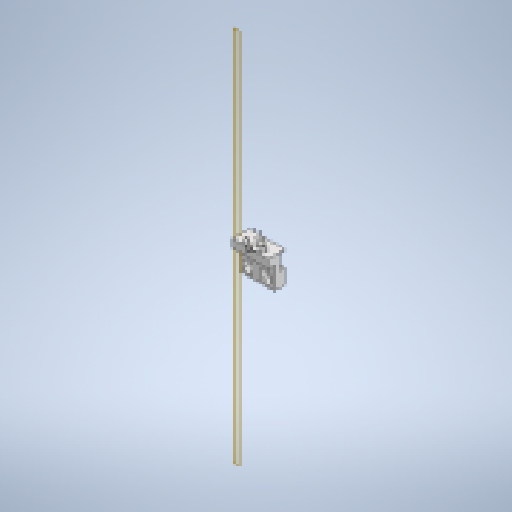
# Autodesk Inventor part: mountingPlate_V7
Saved by Autodesk Inventor 2023 (Build 270158000, 158)
## iProperties
Created: 2023-03-29
Part Number: mountingPlate_V7
Material: Generic
Document SubType Name: Modeling
Designer: shrey
Density: 1 g/cm^3
Appearance: Default
Author: shrey
Autodesk Inventor part; units mm, degrees
(part 1 of 3)
ref_plane "YZ Plane" through (0, 0, 0) normal (1, 0, 0) x (0, 1, 0)
ref_plane "XZ Plane" through (0, 0, 0) normal (0, 1, 0) x (-1, 0, 0)
ref_plane "XY Plane" through (0, 0, 0) normal (0, 0, 1) x (1, 0, 0)
ref_plane "Work Plane1" through (0, 0, 0) normal (0, 0, 1) x (-1, 0, 0)
sketch "Sketch2" plane through (0, 0, 0) normal (0, 0, 1) x (-1, 0, 0)
  spline S0 degree 3 poles (65.1879, 2.1547) (65.1796, 2.1356) (65.1474, 2.0656) (65.0811, 1.9497) (64.9926, 1.84) (64.9127, 1.7608) (64.8451, 1.7103) (64.7759, 1.6619) (64.6996, 1.6258) (64.6221, 1.5923) (64.54, 1.5725) (64.4573, 1.5558) (64.3447, 1.5518) (64.2044, 1.5544) (64.064, 1.5518) (63.9515, 1.5558) (63.8687, 1.5725) (63.7866, 1.5923) (63.7091, 1.6258) (63.6328, 1.6619) (63.5636, 1.7103) (63.4961, 1.7608) (63.4161, 1.84) (63.3277, 1.9497) (63.2437, 2.0964) (63.1793, 2.2524) (63.1317, 2.4143) (63.0866, 2.6344) (63.0241, 2.9083) (62.9282, 3.2316) (62.8191, 3.5506) (62.6977, 3.8651) (62.5657, 4.1753) (62.424, 4.4811) (62.2735, 4.7827) (62.1147, 5.08) (61.8936, 5.4714) (61.7138, 5.7566) (61.594, 5.9467) knots -0.66337 -0.66337 -0.66337 -0.66337 -0.657123 -0.640284 -0.623449 -0.615023 -0.606598 -0.598176 -0.589749 -0.581327 -0.572901 -0.564477 -0.556053 -0.5392 -0.522347 -0.513923 -0.505499 -0.497074 -0.488651 -0.480225 -0.471802 -0.463377 -0.454951 -0.438116 -0.421277 -0.40443 -0.387584 -0.370735 -0.337035 -0.303333 -0.26963 -0.235926 -0.202222 -0.168518 -0.134814 -0.101109 -0.067405 0 0 0 0 construction
  line L0 (61.594, 5.9467) -> (60.5318, 5.9467) construction
  spline S1 degree 3 poles (60.5318, 5.9467) (60.4119, 5.7566) (60.2321, 5.4714) (60.0111, 5.08) (59.8523, 4.7827) (59.7018, 4.4811) (59.5601, 4.1753) (59.428, 3.8651) (59.3066, 3.5506) (59.1976, 3.2316) (59.1016, 2.9083) (59.0392, 2.6344) (58.9941, 2.4143) (58.9464, 2.2524) (58.882, 2.0964) (58.7981, 1.9497) (58.7096, 1.84) (58.6297, 1.7608) (58.5621, 1.7103) (58.4929, 1.6619) (58.4166, 1.6258) (58.3391, 1.5923) (58.257, 1.5725) (58.1743, 1.5558) (58.0617, 1.5518) (57.9214, 1.5544) (57.781, 1.5518) (57.6685, 1.5558) (57.5857, 1.5725) (57.5036, 1.5923) (57.4261, 1.6258) (57.3498, 1.6619) (57.2806, 1.7103) (57.2131, 1.7608) (57.1331, 1.84) (57.0447, 1.9497) (56.9607, 2.0964) (56.8963, 2.2524) (56.8487, 2.4143) (56.8036, 2.6344) (56.7411, 2.9083) (56.6452, 3.2316) (56.5361, 3.5506) (56.4147, 3.8651) (56.2827, 4.1753) (56.141, 4.4811) (55.9905, 4.7827) (55.8317, 5.08) (55.6106, 5.4714) (55.4308, 5.7566) (55.311, 5.9467) knots -1.0784 -1.0784 -1.0784 -1.0784 -1.010995 -0.977291 -0.943586 -0.909882 -0.876178 -0.842474 -0.80877 -0.775067 -0.741365 -0.707665 -0.690816 -0.67397 -0.657123 -0.640284 -0.623449 -0.615023 -0.606598 -0.598176 -0.589749 -0.581327 -0.572901 -0.564477 -0.556053 -0.5392 -0.522347 -0.513923 -0.505499 -0.497074 -0.488651 -0.480225 -0.471802 -0.463377 -0.454951 -0.438116 -0.421277 -0.40443 -0.387584 -0.370735 -0.337035 -0.303333 -0.26963 -0.235926 -0.202222 -0.168518 -0.134814 -0.101109 -0.067405 0 0 0 0 construction
  line L1 (55.311, 5.9467) -> (54.2488, 5.9467) construction
  spline S2 degree 3 poles (54.2488, 5.9467) (54.1289, 5.7566) (53.9491, 5.4714) (53.7281, 5.08) (53.5693, 4.7827) (53.4188, 4.4811) (53.2771, 4.1753) (53.145, 3.8651) (53.0236, 3.5506) (52.9146, 3.2316) (52.8186, 2.9083) (52.7562, 2.6344) (52.7111, 2.4143) (52.6634, 2.2524) (52.599, 2.0964) (52.5151, 1.9497) (52.4266, 1.84) (52.3467, 1.7608) (52.2791, 1.7103) (52.2099, 1.6619) (52.1336, 1.6258) (52.0561, 1.5923) (51.974, 1.5725) (51.8913, 1.5558) (51.7787, 1.5518) (51.6384, 1.5544) (51.498, 1.5518) (51.3855, 1.5558) (51.3027, 1.5725) (51.2206, 1.5923) (51.1431, 1.6258) (51.0668, 1.6619) (50.9976, 1.7103) (50.9301, 1.7608) (50.8501, 1.84) (50.7617, 1.9497) (50.6777, 2.0964) (50.6133, 2.2524) (50.5657, 2.4143) (50.5206, 2.6344) (50.4581, 2.9083) (50.3622, 3.2316) (50.2531, 3.5506) (50.1317, 3.8651) (49.9997, 4.1753) (49.858, 4.4811) (49.7075, 4.7827) (49.5487, 5.08) (49.3276, 5.4714) (49.1478, 5.7566) (49.028, 5.9467) knots -1.0784 -1.0784 -1.0784 -1.0784 -1.010995 -0.977291 -0.943586 -0.909882 -0.876178 -0.842474 -0.80877 -0.775067 -0.741365 -0.707665 -0.690816 -0.67397 -0.657123 -0.640284 -0.623449 -0.615023 -0.606598 -0.598176 -0.589749 -0.581327 -0.572901 -0.564477 -0.556053 -0.5392 -0.522347 -0.513923 -0.505499 -0.497074 -0.488651 -0.480225 -0.471802 -0.463377 -0.454951 -0.438116 -0.421277 -0.40443 -0.387584 -0.370735 -0.337035 -0.303333 -0.26963 -0.235926 -0.202222 -0.168518 -0.134814 -0.101109 -0.067405 0 0 0 0 construction
  line L2 (49.028, 5.9467) -> (47.9658, 5.9467) construction
  spline S3 degree 3 poles (47.9658, 5.9467) (47.8459, 5.7566) (47.6661, 5.4714) (47.4451, 5.08) (47.2863, 4.7827) (47.1358, 4.4811) (46.9941, 4.1753) (46.862, 3.8651) (46.7406, 3.5506) (46.6316, 3.2316) (46.5356, 2.9083) (46.4732, 2.6344) (46.4281, 2.4143) (46.3804, 2.2524) (46.316, 2.0964) (46.2321, 1.9497) (46.1436, 1.84) (46.0637, 1.7608) (45.9961, 1.7103) (45.9269, 1.6619) (45.8506, 1.6258) (45.7731, 1.5923) (45.691, 1.5725) (45.6083, 1.5558) (45.4957, 1.5518) (45.3554, 1.5544) (45.215, 1.5518) (45.1025, 1.5558) (45.0197, 1.5725) (44.9376, 1.5923) (44.8601, 1.6258) (44.7838, 1.6619) (44.7146, 1.7103) (44.6471, 1.7608) (44.5671, 1.84) (44.4787, 1.9497) (44.3947, 2.0964) (44.3303, 2.2524) (44.2827, 2.4143) (44.2376, 2.6344) (44.1751, 2.9083) (44.0792, 3.2316) (43.9701, 3.5506) (43.8487, 3.8651) (43.7167, 4.1753) (43.575, 4.4811) (43.4245, 4.7827) (43.2657, 5.08) (43.0446, 5.4714) (42.8648, 5.7566) (42.745, 5.9467) knots -1.0784 -1.0784 -1.0784 -1.0784 -1.010995 -0.977291 -0.943586 -0.909882 -0.876178 -0.842474 -0.80877 -0.775067 -0.741365 -0.707665 -0.690816 -0.67397 -0.657123 -0.640284 -0.623449 -0.615023 -0.606598 -0.598176 -0.589749 -0.581327 -0.572901 -0.564477 -0.556053 -0.5392 -0.522347 -0.513923 -0.505499 -0.497074 -0.488651 -0.480225 -0.471802 -0.463377 -0.454951 -0.438116 -0.421277 -0.40443 -0.387584 -0.370735 -0.337035 -0.303333 -0.26963 -0.235926 -0.202222 -0.168518 -0.134814 -0.101109 -0.067405 0 0 0 0 construction
  line L3 (42.745, 5.9467) -> (41.6828, 5.9467) construction
  spline S4 degree 3 poles (41.6828, 5.9467) (41.5629, 5.7566) (41.3831, 5.4714) (41.1621, 5.08) (41.0033, 4.7827) (40.8528, 4.4811) (40.7111, 4.1753) (40.579, 3.8651) (40.4576, 3.5506) (40.3486, 3.2316) (40.2526, 2.9083) (40.1902, 2.6344) (40.1451, 2.4143) (40.0974, 2.2524) (40.033, 2.0964) (39.9491, 1.9497) (39.8606, 1.84) (39.7807, 1.7608) (39.7131, 1.7103) (39.6439, 1.6619) (39.5676, 1.6258) (39.4901, 1.5923) (39.408, 1.5725) (39.3253, 1.5558) (39.2127, 1.5518) (39.0724, 1.5544) (38.932, 1.5518) (38.8195, 1.5558) (38.7367, 1.5725) (38.6546, 1.5923) (38.5771, 1.6258) (38.5008, 1.6619) (38.4316, 1.7103) (38.3641, 1.7608) (38.2841, 1.84) (38.1957, 1.9497) (38.1117, 2.0964) (38.0473, 2.2524) (37.9997, 2.4143) (37.9546, 2.6344) (37.8921, 2.9083) (37.7962, 3.2316) (37.6871, 3.5506) (37.5657, 3.8651) (37.4337, 4.1753) (37.292, 4.4811) (37.1415, 4.7827) (36.9827, 5.08) (36.7616, 5.4714) (36.5818, 5.7566) (36.462, 5.9467) knots -1.0784 -1.0784 -1.0784 -1.0784 -1.010995 -0.977291 -0.943586 -0.909882 -0.876178 -0.842474 -0.80877 -0.775067 -0.741365 -0.707665 -0.690816 -0.67397 -0.657123 -0.640284 -0.623449 -0.615023 -0.606598 -0.598176 -0.589749 -0.581327 -0.572901 -0.564477 -0.556053 -0.5392 -0.522347 -0.513923 -0.505499 -0.497074 -0.488651 -0.480225 -0.471802 -0.463377 -0.454951 -0.438116 -0.421277 -0.40443 -0.387584 -0.370735 -0.337035 -0.303333 -0.26963 -0.235926 -0.202222 -0.168518 -0.134814 -0.101109 -0.067405 0 0 0 0 construction
  line L4 (36.462, 5.9467) -> (35.3998, 5.9467) construction
  spline S5 degree 3 poles (35.3998, 5.9467) (35.2799, 5.7566) (35.1001, 5.4714) (34.8791, 5.08) (34.7203, 4.7827) (34.5698, 4.4811) (34.4281, 4.1753) (34.296, 3.8651) (34.1746, 3.5506) (34.0656, 3.2316) (33.9696, 2.9083) (33.9072, 2.6344) (33.8621, 2.4143) (33.8144, 2.2524) (33.75, 2.0964) (33.6661, 1.9497) (33.5776, 1.84) (33.4977, 1.7608) (33.4301, 1.7103) (33.3609, 1.6619) (33.2846, 1.6258) (33.2071, 1.5923) (33.125, 1.5725) (33.0423, 1.5558) (32.9297, 1.5518) (32.7894, 1.5544) (32.649, 1.5518) (32.5365, 1.5558) (32.4537, 1.5725) (32.3716, 1.5923) (32.2941, 1.6258) (32.2178, 1.6619) (32.1486, 1.7103) (32.0811, 1.7608) (32.0011, 1.84) (31.9127, 1.9497) (31.8287, 2.0964) (31.7643, 2.2524) (31.7167, 2.4143) (31.6716, 2.6344) (31.6091, 2.9083) (31.5132, 3.2316) (31.4041, 3.5506) (31.2827, 3.8651) (31.1507, 4.1753) (31.009, 4.4811) (30.8585, 4.7827) (30.6997, 5.08) (30.4786, 5.4714) (30.2988, 5.7566) (30.179, 5.9467) knots -1.0784 -1.0784 -1.0784 -1.0784 -1.010995 -0.977291 -0.943586 -0.909882 -0.876178 -0.842474 -0.80877 -0.775067 -0.741365 -0.707665 -0.690816 -0.67397 -0.657123 -0.640284 -0.623449 -0.615023 -0.606598 -0.598176 -0.589749 -0.581327 -0.572901 -0.564477 -0.556053 -0.5392 -0.522347 -0.513923 -0.505499 -0.497074 -0.488651 -0.480225 -0.471802 -0.463377 -0.454951 -0.438116 -0.421277 -0.40443 -0.387584 -0.370735 -0.337035 -0.303333 -0.26963 -0.235926 -0.202222 -0.168518 -0.134814 -0.101109 -0.067405 0 0 0 0 construction
  line L5 (30.179, 5.9467) -> (29.1168, 5.9467) construction
  spline S6 degree 3 poles (29.1168, 5.9467) (28.9969, 5.7566) (28.8171, 5.4714) (28.5961, 5.08) (28.4373, 4.7827) (28.2868, 4.4811) (28.1451, 4.1753) (28.013, 3.8651) (27.8916, 3.5506) (27.7826, 3.2316) (27.6866, 2.9083) (27.6242, 2.6344) (27.5791, 2.4143) (27.5314, 2.2524) (27.467, 2.0964) (27.3831, 1.9497) (27.2946, 1.84) (27.2147, 1.7608) (27.1471, 1.7103) (27.0779, 1.6619) (27.0016, 1.6258) (26.9241, 1.5923) (26.842, 1.5725) (26.7593, 1.5558) (26.6467, 1.5518) (26.5064, 1.5544) (26.366, 1.5518) (26.2535, 1.5558) (26.1707, 1.5725) (26.0886, 1.5923) (26.0111, 1.6258) (25.9348, 1.6619) (25.8656, 1.7103) (25.7981, 1.7608) (25.7181, 1.84) (25.6297, 1.9497) (25.5457, 2.0964) (25.4813, 2.2524) (25.4337, 2.4143) (25.3886, 2.6344) (25.3261, 2.9083) (25.2302, 3.2316) (25.1211, 3.5506) (24.9997, 3.8651) (24.8677, 4.1753) (24.726, 4.4811) (24.5755, 4.7827) (24.4167, 5.08) (24.1956, 5.4714) (24.0158, 5.7566) (23.896, 5.9467) knots -1.0784 -1.0784 -1.0784 -1.0784 -1.010995 -0.977291 -0.943586 -0.909882 -0.876178 -0.842474 -0.80877 -0.775067 -0.741365 -0.707665 -0.690816 -0.67397 -0.657123 -0.640284 -0.623449 -0.615023 -0.606598 -0.598176 -0.589749 -0.581327 -0.572901 -0.564477 -0.556053 -0.5392 -0.522347 -0.513923 -0.505499 -0.497074 -0.488651 -0.480225 -0.471802 -0.463377 -0.454951 -0.438116 -0.421277 -0.40443 -0.387584 -0.370735 -0.337035 -0.303333 -0.26963 -0.235926 -0.202222 -0.168518 -0.134814 -0.101109 -0.067405 0 0 0 0 construction
  line L6 (23.896, 5.9467) -> (22.8338, 5.9467) construction
  spline S7 degree 3 poles (22.8338, 5.9467) (22.7139, 5.7566) (22.5341, 5.4714) (22.3131, 5.08) (22.1543, 4.7827) (22.0038, 4.4811) (21.8621, 4.1753) (21.73, 3.8651) (21.6086, 3.5506) (21.4996, 3.2316) (21.4036, 2.9083) (21.3412, 2.6344) (21.2961, 2.4143) (21.2484, 2.2524) (21.184, 2.0964) (21.1001, 1.9497) (21.0116, 1.84) (20.9317, 1.7608) (20.8641, 1.7103) (20.7949, 1.6619) (20.7186, 1.6258) (20.6411, 1.5923) (20.559, 1.5725) (20.4763, 1.5558) (20.3637, 1.5518) (20.2234, 1.5544) (20.083, 1.5518) (19.9705, 1.5558) (19.8877, 1.5725) (19.8056, 1.5923) (19.7281, 1.6258) (19.6518, 1.6619) (19.5826, 1.7103) (19.5151, 1.7608) (19.4351, 1.84) (19.3467, 1.9497) (19.2627, 2.0964) (19.1983, 2.2524) (19.1507, 2.4143) (19.1056, 2.6344) (19.0431, 2.9083) (18.9472, 3.2316) (18.8381, 3.5506) (18.7167, 3.8651) (18.5847, 4.1753) (18.443, 4.4811) (18.2925, 4.7827) (18.1337, 5.08) (17.9126, 5.4714) (17.7328, 5.7566) (17.613, 5.9467) knots -1.0784 -1.0784 -1.0784 -1.0784 -1.010995 -0.977291 -0.943586 -0.909882 -0.876178 -0.842474 -0.80877 -0.775067 -0.741365 -0.707665 -0.690816 -0.67397 -0.657123 -0.640284 -0.623449 -0.615023 -0.606598 -0.598176 -0.589749 -0.581327 -0.572901 -0.564477 -0.556053 -0.5392 -0.522347 -0.513923 -0.505499 -0.497074 -0.488651 -0.480225 -0.471802 -0.463377 -0.454951 -0.438116 -0.421277 -0.40443 -0.387584 -0.370735 -0.337035 -0.303333 -0.26963 -0.235926 -0.202222 -0.168518 -0.134814 -0.101109 -0.067405 0 0 0 0 construction
  line L7 (17.613, 5.9467) -> (16.5508, 5.9467) construction
  spline S8 degree 3 poles (16.5508, 5.9467) (16.4309, 5.7566) (16.2511, 5.4714) (16.0301, 5.08) (15.8713, 4.7827) (15.7208, 4.4811) (15.5791, 4.1753) (15.447, 3.8651) (15.3256, 3.5506) (15.2166, 3.2316) (15.1206, 2.9083) (15.0582, 2.6344) (15.0131, 2.4143) (14.9654, 2.2524) (14.901, 2.0964) (14.8171, 1.9497) (14.7286, 1.84) (14.6487, 1.7608) (14.5811, 1.7103) (14.5119, 1.6619) (14.4356, 1.6258) (14.3581, 1.5923) (14.276, 1.5725) (14.1933, 1.5558) (14.0807, 1.5518) (13.9404, 1.5544) (13.8, 1.5518) (13.6875, 1.5558) (13.6047, 1.5725) (13.5226, 1.5923) (13.4451, 1.6258) (13.3688, 1.6619) (13.2996, 1.7103) (13.2321, 1.7608) (13.1521, 1.84) (13.0637, 1.9497) (12.9797, 2.0964) (12.9153, 2.2524) (12.8677, 2.4143) (12.8226, 2.6344) (12.7601, 2.9083) (12.6642, 3.2316) (12.5551, 3.5506) (12.4337, 3.8651) (12.3017, 4.1753) (12.16, 4.4811) (12.0095, 4.7827) (11.8507, 5.08) (11.6296, 5.4714) (11.4498, 5.7566) (11.33, 5.9467) knots -1.0784 -1.0784 -1.0784 -1.0784 -1.010995 -0.977291 -0.943586 -0.909882 -0.876178 -0.842474 -0.80877 -0.775067 -0.741365 -0.707665 -0.690816 -0.67397 -0.657123 -0.640284 -0.623449 -0.615023 -0.606598 -0.598176 -0.589749 -0.581327 -0.572901 -0.564477 -0.556053 -0.5392 -0.522347 -0.513923 -0.505499 -0.497074 -0.488651 -0.480225 -0.471802 -0.463377 -0.454951 -0.438116 -0.421277 -0.40443 -0.387584 -0.370735 -0.337035 -0.303333 -0.26963 -0.235926 -0.202222 -0.168518 -0.134814 -0.101109 -0.067405 0 0 0 0 construction
  line L8 (11.33, 5.9467) -> (10.2678, 5.9467) construction
  spline S9 degree 3 poles (10.2678, 5.9467) (10.1479, 5.7566) (9.9681, 5.4714) (9.7471, 5.08) (9.5883, 4.7827) (9.4378, 4.4811) (9.2961, 4.1753) (9.164, 3.8651) (9.0426, 3.5506) (8.9336, 3.2316) (8.8376, 2.9083) (8.7752, 2.6344) (8.7301, 2.4143) (8.6824, 2.2524) (8.618, 2.0964) (8.5341, 1.9497) (8.4456, 1.84) (8.3657, 1.7608) (8.2981, 1.7103) (8.2289, 1.6619) (8.1526, 1.6258) (8.0751, 1.5923) (7.993, 1.5725) (7.9103, 1.5558) (7.7977, 1.5518) (7.6574, 1.5544) (7.517, 1.5518) (7.4045, 1.5558) (7.3217, 1.5725) (7.2396, 1.5923) (7.1621, 1.6258) (7.0858, 1.6619) (7.0166, 1.7103) (6.9491, 1.7608) (6.8691, 1.84) (6.7807, 1.9497) (6.6967, 2.0964) (6.6323, 2.2524) (6.5847, 2.4143) (6.5396, 2.6344) (6.4771, 2.9083) (6.3812, 3.2316) (6.2721, 3.5506) (6.1507, 3.8651) (6.0187, 4.1753) (5.877, 4.4811) (5.7265, 4.7827) (5.5677, 5.08) (5.3466, 5.4714) (5.1668, 5.7566) (5.047, 5.9467) knots -1.0784 -1.0784 -1.0784 -1.0784 -1.010995 -0.977291 -0.943586 -0.909882 -0.876178 -0.842474 -0.80877 -0.775067 -0.741365 -0.707665 -0.690816 -0.67397 -0.657123 -0.640284 -0.623449 -0.615023 -0.606598 -0.598176 -0.589749 -0.581327 -0.572901 -0.564477 -0.556053 -0.5392 -0.522347 -0.513923 -0.505499 -0.497074 -0.488651 -0.480225 -0.471802 -0.463377 -0.454951 -0.438116 -0.421277 -0.40443 -0.387584 -0.370735 -0.337035 -0.303333 -0.26963 -0.235926 -0.202222 -0.168518 -0.134814 -0.101109 -0.067405 0 0 0 0 construction
  line L9 (5.047, 5.9467) -> (3.9848, 5.9467) construction
  spline S10 degree 3 poles (3.9848, 5.9467) (3.8649, 5.7566) (3.6851, 5.4714) (3.4641, 5.08) (3.3053, 4.7827) (3.1548, 4.4811) (3.0131, 4.1753) (2.881, 3.8651) (2.7596, 3.5506) (2.6506, 3.2316) (2.5546, 2.9083) (2.4922, 2.6344) (2.4471, 2.4143) (2.3994, 2.2524) (2.335, 2.0964) (2.2511, 1.9497) (2.1626, 1.84) (2.0827, 1.7608) (2.0151, 1.7103) (1.9459, 1.6619) (1.8696, 1.6258) (1.7921, 1.5923) (1.71, 1.5725) (1.6273, 1.5558) (1.5147, 1.5518) (1.3744, 1.5544) (1.234, 1.5518) (1.1215, 1.5558) (1.0387, 1.5725) (0.9566, 1.5923) (0.8791, 1.6258) (0.8028, 1.6619) (0.7336, 1.7103) (0.6661, 1.7608) (0.5861, 1.84) (0.4977, 1.9497) (0.4137, 2.0964) (0.3493, 2.2524) (0.3017, 2.4143) (0.2566, 2.6344) (0.1941, 2.9083) (0.0982, 3.2316) (-0.0109, 3.5506) (-0.1323, 3.8651) (-0.2643, 4.1753) (-0.406, 4.4811) (-0.5565, 4.7827) (-0.7153, 5.08) (-0.9364, 5.4714) (-1.1162, 5.7566) (-1.236, 5.9467) knots -1.0784 -1.0784 -1.0784 -1.0784 -1.010995 -0.977291 -0.943586 -0.909882 -0.876178 -0.842474 -0.80877 -0.775067 -0.741365 -0.707665 -0.690816 -0.67397 -0.657123 -0.640284 -0.623449 -0.615023 -0.606598 -0.598176 -0.589749 -0.581327 -0.572901 -0.564477 -0.556053 -0.5392 -0.522347 -0.513923 -0.505499 -0.497074 -0.488651 -0.480225 -0.471802 -0.463377 -0.454951 -0.438116 -0.421277 -0.40443 -0.387584 -0.370735 -0.337035 -0.303333 -0.26963 -0.235926 -0.202222 -0.168518 -0.134814 -0.101109 -0.067405 0 0 0 0 construction
  line L10 (-1.236, 5.9467) -> (-2.2982, 5.9467) construction
  spline S11 degree 3 poles (-2.2982, 5.9467) (-2.4181, 5.7566) (-2.5979, 5.4714) (-2.8189, 5.08) (-2.9777, 4.7827) (-3.1282, 4.4811) (-3.2699, 4.1753) (-3.402, 3.8651) (-3.5234, 3.5506) (-3.6324, 3.2316) (-3.7284, 2.9083) (-3.7908, 2.6344) (-3.8359, 2.4143) (-3.8836, 2.2524) (-3.948, 2.0964) (-4.0319, 1.9497) (-4.1204, 1.84) (-4.2003, 1.7608) (-4.2679, 1.7103) (-4.3371, 1.6619) (-4.4134, 1.6258) (-4.4909, 1.5923) (-4.573, 1.5725) (-4.6557, 1.5558) (-4.7683, 1.5518) (-4.9086, 1.5544) (-5.049, 1.5518) (-5.1615, 1.5558) (-5.2443, 1.5725) (-5.3264, 1.5923) (-5.4039, 1.6258) (-5.4802, 1.6619) (-5.5494, 1.7103) (-5.6169, 1.7608) (-5.6969, 1.84) (-5.7853, 1.9497) (-5.8693, 2.0964) (-5.9337, 2.2524) (-5.9813, 2.4143) (-6.0264, 2.6344) (-6.0889, 2.9083) (-6.1848, 3.2316) (-6.2939, 3.5506) (-6.4153, 3.8651) (-6.5473, 4.1753) (-6.689, 4.4811) (-6.8395, 4.7827) (-6.9983, 5.08) (-7.2194, 5.4714) (-7.3992, 5.7566) (-7.519, 5.9467) knots -1.0784 -1.0784 -1.0784 -1.0784 -1.010995 -0.977291 -0.943586 -0.909882 -0.876178 -0.842474 -0.80877 -0.775067 -0.741365 -0.707665 -0.690816 -0.67397 -0.657123 -0.640284 -0.623449 -0.615023 -0.606598 -0.598176 -0.589749 -0.581327 -0.572901 -0.564477 -0.556053 -0.5392 -0.522347 -0.513923 -0.505499 -0.497074 -0.488651 -0.480225 -0.471802 -0.463377 -0.454951 -0.438116 -0.421277 -0.40443 -0.387584 -0.370735 -0.337035 -0.303333 -0.26963 -0.235926 -0.202222 -0.168518 -0.134814 -0.101109 -0.067405 0 0 0 0 construction
  line L11 (-7.519, 5.9467) -> (-8.5812, 5.9467) construction
  spline S12 degree 3 poles (-8.5812, 5.9467) (-8.7011, 5.7566) (-8.8809, 5.4714) (-9.1019, 5.08) (-9.2607, 4.7827) (-9.4112, 4.4811) (-9.5529, 4.1753) (-9.685, 3.8651) (-9.8064, 3.5506) (-9.9154, 3.2316) (-10.0114, 2.9083) (-10.0738, 2.6344) (-10.1189, 2.4143) (-10.1666, 2.2524) (-10.231, 2.0964) (-10.3149, 1.9497) (-10.4034, 1.84) (-10.4833, 1.7608) (-10.5509, 1.7103) (-10.6201, 1.6619) (-10.6964, 1.6258) (-10.7739, 1.5923) (-10.856, 1.5725) (-10.9387, 1.5558) (-11.0513, 1.5518) (-11.1916, 1.5544) (-11.332, 1.5518) (-11.4445, 1.5558) (-11.5273, 1.5725) (-11.6094, 1.5923) (-11.6869, 1.6258) (-11.7632, 1.6619) (-11.8324, 1.7103) (-11.8999, 1.7608) (-11.9799, 1.84) (-12.0683, 1.9497) (-12.1523, 2.0964) (-12.2167, 2.2524) (-12.2643, 2.4143) (-12.3094, 2.6344) (-12.3719, 2.9083) (-12.4678, 3.2316) (-12.5769, 3.5506) (-12.6983, 3.8651) (-12.8303, 4.1753) (-12.972, 4.4811) (-13.1225, 4.7827) (-13.2813, 5.08) (-13.5024, 5.4714) (-13.6822, 5.7566) (-13.802, 5.9467) knots -1.0784 -1.0784 -1.0784 -1.0784 -1.010995 -0.977291 -0.943586 -0.909882 -0.876178 -0.842474 -0.80877 -0.775067 -0.741365 -0.707665 -0.690816 -0.67397 -0.657123 -0.640284 -0.623449 -0.615023 -0.606598 -0.598176 -0.589749 -0.581327 -0.572901 -0.564477 -0.556053 -0.5392 -0.522347 -0.513923 -0.505499 -0.497074 -0.488651 -0.480225 -0.471802 -0.463377 -0.454951 -0.438116 -0.421277 -0.40443 -0.387584 -0.370735 -0.337035 -0.303333 -0.26963 -0.235926 -0.202222 -0.168518 -0.134814 -0.101109 -0.067405 0 0 0 0 construction
  line L12 (-13.802, 5.9467) -> (-14.8642, 5.9467) construction
  spline S13 degree 3 poles (-14.8642, 5.9467) (-14.9841, 5.7566) (-15.1639, 5.4714) (-15.3849, 5.08) (-15.5437, 4.7827) (-15.6942, 4.4811) (-15.8359, 4.1753) (-15.968, 3.8651) (-16.0894, 3.5506) (-16.1984, 3.2316) (-16.2944, 2.9083) (-16.3568, 2.6344) (-16.4019, 2.4143) (-16.4496, 2.2524) (-16.514, 2.0964) (-16.5979, 1.9497) (-16.6864, 1.84) (-16.7663, 1.7608) (-16.8339, 1.7103) (-16.9031, 1.6619) (-16.9794, 1.6258) (-17.0569, 1.5923) (-17.139, 1.5725) (-17.2217, 1.5558) (-17.3343, 1.5518) (-17.4746, 1.5544) (-17.615, 1.5518) (-17.7275, 1.5558) (-17.8103, 1.5725) (-17.8924, 1.5923) (-17.9699, 1.6258) (-18.0462, 1.6619) (-18.1154, 1.7103) (-18.1829, 1.7608) (-18.2629, 1.84) (-18.3513, 1.9497) (-18.4353, 2.0964) (-18.4997, 2.2524) (-18.5473, 2.4143) (-18.5924, 2.6344) (-18.6549, 2.9083) (-18.7508, 3.2316) (-18.8599, 3.5506) (-18.9813, 3.8651) (-19.1133, 4.1753) (-19.255, 4.4811) (-19.4055, 4.7827) (-19.5643, 5.08) (-19.7854, 5.4714) (-19.9652, 5.7566) (-20.085, 5.9467) knots -1.0784 -1.0784 -1.0784 -1.0784 -1.010995 -0.977291 -0.943586 -0.909882 -0.876178 -0.842474 -0.80877 -0.775067 -0.741365 -0.707665 -0.690816 -0.67397 -0.657123 -0.640284 -0.623449 -0.615023 -0.606598 -0.598176 -0.589749 -0.581327 -0.572901 -0.564477 -0.556053 -0.5392 -0.522347 -0.513923 -0.505499 -0.497074 -0.488651 -0.480225 -0.471802 -0.463377 -0.454951 -0.438116 -0.421277 -0.40443 -0.387584 -0.370735 -0.337035 -0.303333 -0.26963 -0.235926 -0.202222 -0.168518 -0.134814 -0.101109 -0.067405 0 0 0 0 construction
  line L13 (-20.085, 5.9467) -> (-21.1472, 5.9467) construction
  spline S14 degree 3 poles (-21.1472, 5.9467) (-21.2671, 5.7566) (-21.4469, 5.4714) (-21.6679, 5.08) (-21.8267, 4.7827) (-21.9772, 4.4811) (-22.1189, 4.1753) (-22.251, 3.8651) (-22.3724, 3.5506) (-22.4814, 3.2316) (-22.5774, 2.9083) (-22.6398, 2.6344) (-22.6849, 2.4143) (-22.7326, 2.2524) (-22.797, 2.0964) (-22.8809, 1.9497) (-22.9694, 1.84) (-23.0493, 1.7608) (-23.1169, 1.7103) (-23.1861, 1.6619) (-23.2624, 1.6258) (-23.3399, 1.5923) (-23.422, 1.5725) (-23.5047, 1.5558) (-23.6173, 1.5518) (-23.7576, 1.5544) (-23.898, 1.5518) (-24.0105, 1.5558) (-24.0933, 1.5725) (-24.1754, 1.5923) (-24.2529, 1.6258) (-24.3292, 1.6619) (-24.3984, 1.7103) (-24.4659, 1.7608) (-24.5459, 1.84) (-24.6343, 1.9497) (-24.7183, 2.0964) (-24.7827, 2.2524) (-24.8303, 2.4143) (-24.8754, 2.6344) (-24.9379, 2.9083) (-25.0338, 3.2316) (-25.1429, 3.5506) (-25.2643, 3.8651) (-25.3963, 4.1753) (-25.538, 4.4811) (-25.6885, 4.7827) (-25.8473, 5.08) (-26.0684, 5.4714) (-26.2482, 5.7566) (-26.368, 5.9467) knots -1.0784 -1.0784 -1.0784 -1.0784 -1.010995 -0.977291 -0.943586 -0.909882 -0.876178 -0.842474 -0.80877 -0.775067 -0.741365 -0.707665 -0.690816 -0.67397 -0.657123 -0.640284 -0.623449 -0.615023 -0.606598 -0.598176 -0.589749 -0.581327 -0.572901 -0.564477 -0.556053 -0.5392 -0.522347 -0.513923 -0.505499 -0.497074 -0.488651 -0.480225 -0.471802 -0.463377 -0.454951 -0.438116 -0.421277 -0.40443 -0.387584 -0.370735 -0.337035 -0.303333 -0.26963 -0.235926 -0.202222 -0.168518 -0.134814 -0.101109 -0.067405 0 0 0 0 construction
  line L14 (-26.368, 5.9467) -> (-27.4302, 5.9467) construction
  spline S15 degree 3 poles (-27.4302, 5.9467) (-27.5501, 5.7566) (-27.7299, 5.4714) (-27.9509, 5.08) (-28.1097, 4.7827) (-28.2602, 4.4811) (-28.4019, 4.1753) (-28.534, 3.8651) (-28.6554, 3.5506) (-28.7644, 3.2316) (-28.8604, 2.9083) (-28.9228, 2.6344) (-28.9679, 2.4143) (-29.0156, 2.2524) (-29.08, 2.0964) (-29.1639, 1.9497) (-29.2524, 1.84) (-29.3323, 1.7608) (-29.3999, 1.7103) (-29.4691, 1.6619) (-29.5454, 1.6258) (-29.6229, 1.5923) (-29.705, 1.5725) (-29.7877, 1.5558) (-29.9003, 1.5518) (-30.0406, 1.5544) (-30.181, 1.5518) (-30.2935, 1.5558) (-30.3763, 1.5725) (-30.4584, 1.5923) (-30.5359, 1.6258) (-30.6122, 1.6619) (-30.6814, 1.7103) (-30.7489, 1.7608) (-30.8289, 1.84) (-30.9173, 1.9497) (-31.0013, 2.0964) (-31.0657, 2.2524) (-31.1133, 2.4143) (-31.1584, 2.6344) (-31.2209, 2.9083) (-31.3168, 3.2316) (-31.4259, 3.5506) (-31.5473, 3.8651) (-31.6793, 4.1753) (-31.821, 4.4811) (-31.9715, 4.7827) (-32.1303, 5.08) (-32.3514, 5.4714) (-32.5312, 5.7566) (-32.651, 5.9467) knots -1.0784 -1.0784 -1.0784 -1.0784 -1.010995 -0.977291 -0.943586 -0.909882 -0.876178 -0.842474 -0.80877 -0.775067 -0.741365 -0.707665 -0.690816 -0.67397 -0.657123 -0.640284 -0.623449 -0.615023 -0.606598 -0.598176 -0.589749 -0.581327 -0.572901 -0.564477 -0.556053 -0.5392 -0.522347 -0.513923 -0.505499 -0.497074 -0.488651 -0.480225 -0.471802 -0.463377 -0.454951 -0.438116 -0.421277 -0.40443 -0.387584 -0.370735 -0.337035 -0.303333 -0.26963 -0.235926 -0.202222 -0.168518 -0.134814 -0.101109 -0.067405 0 0 0 0 construction
  line L15 (-32.651, 5.9467) -> (-33.7132, 5.9467) construction
  spline S16 degree 3 poles (-33.7132, 5.9467) (-33.8331, 5.7566) (-34.0129, 5.4714) (-34.2339, 5.08) (-34.3927, 4.7827) (-34.5432, 4.4811) (-34.6849, 4.1753) (-34.817, 3.8651) (-34.9384, 3.5506) (-35.0474, 3.2316) (-35.1434, 2.9083) (-35.2058, 2.6344) (-35.2509, 2.4143) (-35.2986, 2.2524) (-35.363, 2.0964) (-35.4469, 1.9497) (-35.5354, 1.84) (-35.6153, 1.7608) (-35.6829, 1.7103) (-35.7521, 1.6619) (-35.8284, 1.6258) (-35.9059, 1.5923) (-35.988, 1.5725) (-36.0707, 1.5558) (-36.1833, 1.5518) (-36.3236, 1.5544) (-36.464, 1.5518) (-36.5765, 1.5558) (-36.6593, 1.5725) (-36.7414, 1.5923) (-36.8189, 1.6258) (-36.8952, 1.6619) (-36.9644, 1.7103) (-37.0319, 1.7608) (-37.1119, 1.84) (-37.2003, 1.9497) (-37.2843, 2.0964) (-37.3487, 2.2524) (-37.3963, 2.4143) (-37.4414, 2.6344) (-37.5039, 2.9083) (-37.5998, 3.2316) (-37.7089, 3.5506) (-37.8303, 3.8651) (-37.9623, 4.1753) (-38.104, 4.4811) (-38.2545, 4.7827) (-38.4133, 5.08) (-38.6344, 5.4714) (-38.8142, 5.7566) (-38.934, 5.9467) knots -1.0784 -1.0784 -1.0784 -1.0784 -1.010995 -0.977291 -0.943586 -0.909882 -0.876178 -0.842474 -0.80877 -0.775067 -0.741365 -0.707665 -0.690816 -0.67397 -0.657123 -0.640284 -0.623449 -0.615023 -0.606598 -0.598176 -0.589749 -0.581327 -0.572901 -0.564477 -0.556053 -0.5392 -0.522347 -0.513923 -0.505499 -0.497074 -0.488651 -0.480225 -0.471802 -0.463377 -0.454951 -0.438116 -0.421277 -0.40443 -0.387584 -0.370735 -0.337035 -0.303333 -0.26963 -0.235926 -0.202222 -0.168518 -0.134814 -0.101109 -0.067405 0 0 0 0 construction
  line L16 (-38.934, 5.9467) -> (-39.9962, 5.9467) construction
  spline S17 degree 3 poles (-39.9962, 5.9467) (-40.1161, 5.7566) (-40.2959, 5.4714) (-40.5169, 5.08) (-40.6757, 4.7827) (-40.8262, 4.4811) (-40.9679, 4.1753) (-41.1, 3.8651) (-41.2214, 3.5506) (-41.3304, 3.2316) (-41.4264, 2.9083) (-41.4888, 2.6344) (-41.5339, 2.4143) (-41.5816, 2.2524) (-41.646, 2.0964) (-41.7299, 1.9497) (-41.8184, 1.84) (-41.8983, 1.7608) (-41.9659, 1.7103) (-42.0351, 1.6619) (-42.1114, 1.6258) (-42.1889, 1.5923) (-42.271, 1.5725) (-42.3537, 1.5558) (-42.4663, 1.5518) (-42.6066, 1.5544) (-42.747, 1.5518) (-42.8595, 1.5558) (-42.9423, 1.5725) (-43.0244, 1.5923) (-43.1019, 1.6258) (-43.1782, 1.6619) (-43.2474, 1.7103) (-43.3149, 1.7608) (-43.3949, 1.84) (-43.4833, 1.9497) (-43.5673, 2.0964) (-43.6317, 2.2524) (-43.6793, 2.4143) (-43.7244, 2.6344) (-43.7869, 2.9083) (-43.8828, 3.2316) (-43.9919, 3.5506) (-44.1133, 3.8651) (-44.2453, 4.1753) (-44.387, 4.4811) (-44.5375, 4.7827) (-44.6963, 5.08) (-44.9174, 5.4714) (-45.0972, 5.7566) (-45.217, 5.9467) knots -1.0784 -1.0784 -1.0784 -1.0784 -1.010995 -0.977291 -0.943586 -0.909882 -0.876178 -0.842474 -0.80877 -0.775067 -0.741365 -0.707665 -0.690816 -0.67397 -0.657123 -0.640284 -0.623449 -0.615023 -0.606598 -0.598176 -0.589749 -0.581327 -0.572901 -0.564477 -0.556053 -0.5392 -0.522347 -0.513923 -0.505499 -0.497074 -0.488651 -0.480225 -0.471802 -0.463377 -0.454951 -0.438116 -0.421277 -0.40443 -0.387584 -0.370735 -0.337035 -0.303333 -0.26963 -0.235926 -0.202222 -0.168518 -0.134814 -0.101109 -0.067405 0 0 0 0 construction
  line L17 (-45.217, 5.9467) -> (-46.2792, 5.9467) construction
  spline S18 degree 3 poles (-46.2792, 5.9467) (-46.3991, 5.7566) (-46.5789, 5.4714) (-46.7999, 5.08) (-46.9587, 4.7827) (-47.1092, 4.4811) (-47.2509, 4.1753) (-47.383, 3.8651) (-47.5044, 3.5506) (-47.6134, 3.2316) (-47.7094, 2.9083) (-47.7718, 2.6344) (-47.8169, 2.4143) (-47.8646, 2.2524) (-47.929, 2.0964) (-48.0129, 1.9497) (-48.1014, 1.84) (-48.1813, 1.7608) (-48.2489, 1.7103) (-48.3181, 1.6619) (-48.3944, 1.6258) (-48.4719, 1.5923) (-48.554, 1.5725) (-48.6367, 1.5558) (-48.7493, 1.5518) (-48.8896, 1.5544) (-49.03, 1.5518) (-49.1425, 1.5558) (-49.2253, 1.5725) (-49.3074, 1.5923) (-49.3849, 1.6258) (-49.4612, 1.6619) (-49.5304, 1.7103) (-49.5979, 1.7608) (-49.6779, 1.84) (-49.7663, 1.9497) (-49.8503, 2.0964) (-49.9147, 2.2524) (-49.9623, 2.4143) (-50.0074, 2.6344) (-50.0699, 2.9083) (-50.1658, 3.2316) (-50.2749, 3.5506) (-50.3963, 3.8651) (-50.5283, 4.1753) (-50.67, 4.4811) (-50.8205, 4.7827) (-50.9793, 5.08) (-51.2004, 5.4714) (-51.3802, 5.7566) (-51.5, 5.9467) knots -1.0784 -1.0784 -1.0784 -1.0784 -1.010995 -0.977291 -0.943586 -0.909882 -0.876178 -0.842474 -0.80877 -0.775067 -0.741365 -0.707665 -0.690816 -0.67397 -0.657123 -0.640284 -0.623449 -0.615023 -0.606598 -0.598176 -0.589749 -0.581327 -0.572901 -0.564477 -0.556053 -0.5392 -0.522347 -0.513923 -0.505499 -0.497074 -0.488651 -0.480225 -0.471802 -0.463377 -0.454951 -0.438116 -0.421277 -0.40443 -0.387584 -0.370735 -0.337035 -0.303333 -0.26963 -0.235926 -0.202222 -0.168518 -0.134814 -0.101109 -0.067405 0 0 0 0 construction
  line L18 (-51.5, 5.9467) -> (-51.5, -5.9467) construction
  line L19 (-51.5, -5.9467) -> (65.1879, -5.9467) construction
  line L20 (65.1879, -5.9467) -> (65.1879, 2.1547) construction
  arc A0 (-6.5, 26.4467) -> (-21.5, 26.4467) centre (-14, 19.8323) ccw construction
  line L21 (-6.5, 13.4467) -> (-6.5, 26.4467) construction
  arc A1 (-21.5, 13.4467) -> (-6.5, 13.4467) centre (-14, 20.0611) ccw construction
  line L22 (-21.5, 26.4467) -> (-21.5, 13.4467) construction
  arc A2 (-56.5, 13.4467) -> (-41.5, 13.4467) centre (-49, 20.0611) ccw construction
  line L23 (-56.5, 26.4467) -> (-56.5, 13.4467) construction
  arc A3 (-41.5, 26.4467) -> (-56.5, 26.4467) centre (-49, 19.8323) ccw construction
  line L24 (-41.5, 13.4467) -> (-41.5, 26.4467) construction
  spline S19 degree 3 poles (-18.1738, 36.4263) (-18.2175, 36.3004) (-18.305, 36.0485) (-18.4143, 35.6636) (-18.506, 35.2743) (-18.5766, 34.8805) (-18.6238, 34.4832) (-18.6405, 34.15) (-18.6374, 33.8833) (-18.6248, 33.6838) (-18.603, 33.4847) (-18.572, 33.355) (-18.5564, 33.2902) knots 0 0 0 0 0.125009 0.250019 0.375028 0.500033 0.625034 0.750027 0.812532 0.875036 0.937535 1 1 1 1 construction
  spline S20 degree 3 poles (-18.5564, 33.2902) (-18.5238, 33.2017) (-18.4747, 33.069) (-18.4248, 32.8871) (-18.3972, 32.7484) (-18.3764, 32.6084) (-18.3688, 32.467) (-18.3701, 32.3255) (-18.3871, 32.1848) (-18.4186, 32.0467) (-18.4669, 31.9134) (-18.5324, 31.7877) (-18.6151, 31.6723) (-18.7142, 31.5709) (-18.8278, 31.4856) (-18.9543, 31.4216) (-19.0846, 31.3669) (-19.2125, 31.3067) (-19.3447, 31.2555) (-19.484, 31.2282) (-19.6258, 31.2223) (-19.7668, 31.2381) (-19.9041, 31.2736) (-20.0354, 31.3269) (-20.1592, 31.3958) (-20.2751, 31.4773) (-20.3812, 31.5711) (-20.4811, 31.6713) (-20.5712, 31.7804) (-20.6558, 31.8938) (-20.7576, 32.0526) (-20.8234, 32.1779) (-20.8673, 32.2613) knots 0 0 0 0 0.062498 0.093754 0.125008 0.156267 0.187517 0.21877 0.250029 0.281282 0.312529 0.343776 0.37503 0.406277 0.437515 0.468744 0.5 0.531256 0.562485 0.593723 0.62497 0.656224 0.687471 0.718718 0.749971 0.78123 0.812483 0.843733 0.874992 0.906246 0.937502 1 1 1 1 construction
  spline S21 degree 3 poles (-20.8673, 32.2613) (-20.9051, 32.3162) (-20.9807, 32.4261) (-21.1141, 32.5755) (-21.2539, 32.7184) (-21.45, 32.8991) (-21.7088, 33.1097) (-22.0356, 33.3404) (-22.3755, 33.5514) (-22.7263, 33.7438) (-23.0854, 33.9202) (-23.3311, 34.0237) (-23.454, 34.0754) knots 0 0 0 0 0.062465 0.124964 0.187468 0.249973 0.374966 0.499967 0.624972 0.749981 0.874991 1 1 1 1 construction
  arc A4 (-23.454, 34.0754) -> (-24.5158, 33.304) centre (-14, 19.9467) ccw construction
  spline S22 degree 3 poles (-24.5158, 33.304) (-24.5046, 33.1711) (-24.4821, 32.9054) (-24.4253, 32.5094) (-24.3507, 32.1164) (-24.255, 31.7279) (-24.1366, 31.3457) (-24.0163, 31.0346) (-23.905, 30.7923) (-23.8124, 30.6151) (-23.7115, 30.4421) (-23.6304, 30.3362) (-23.5898, 30.2833) knots 0 0 0 0 0.125009 0.250019 0.375028 0.500033 0.625034 0.750027 0.812532 0.875036 0.937535 1 1 1 1 construction
  spline S23 degree 3 poles (-23.5898, 30.2833) (-23.524, 30.2158) (-23.4252, 30.1145) (-23.3056, 29.9686) (-23.2239, 29.8531) (-23.148, 29.7336) (-23.0836, 29.6077) (-23.0272, 29.4778) (-22.9855, 29.3424) (-22.9582, 29.2034) (-22.948, 29.062) (-22.9568, 28.9205) (-22.9853, 28.7815) (-23.0347, 28.6485) (-23.1037, 28.5244) (-23.1933, 28.4145) (-23.2901, 28.3115) (-23.3824, 28.2045) (-23.4823, 28.1039) (-23.5985, 28.0223) (-23.7256, 27.9593) (-23.8609, 27.9164) (-24.0007, 27.8929) (-24.1424, 27.8882) (-24.2835, 27.9008) (-24.4225, 27.9282) (-24.5576, 27.9706) (-24.6896, 28.0216) (-24.8163, 28.0846) (-24.9397, 28.1537) (-25.0973, 28.2574) (-25.2084, 28.3451) (-25.2824, 28.4035) knots 0 0 0 0 0.062498 0.093754 0.125008 0.156267 0.187517 0.21877 0.250029 0.281282 0.312529 0.343776 0.37503 0.406277 0.437515 0.468744 0.5 0.531256 0.562485 0.593723 0.62497 0.656224 0.687471 0.718718 0.749971 0.78123 0.812483 0.843733 0.874992 0.906246 0.937502 1 1 1 1 construction
  spline S24 degree 3 poles (-25.2824, 28.4035) (-25.3393, 28.4383) (-25.4531, 28.5079) (-25.6356, 28.5901) (-25.8215, 28.6638) (-26.0742, 28.7491) (-26.3962, 28.8362) (-26.7886, 28.9141) (-27.185, 28.9686) (-27.5836, 29.0017) (-27.9835, 29.0168) (-28.25, 29.0114) (-28.3833, 29.0087) knots 0 0 0 0 0.062465 0.124964 0.187468 0.249973 0.374966 0.499967 0.624972 0.749981 0.874991 1 1 1 1 construction
  arc A5 (-28.3833, 29.0087) -> (-29.0396, 27.872) centre (-14, 19.9467) ccw construction
  spline S25 degree 3 poles (-29.0396, 27.872) (-28.9753, 27.7552) (-28.8467, 27.5217) (-28.6337, 27.1829) (-28.4057, 26.8542) (-28.1603, 26.5383) (-27.8967, 26.2373) (-27.6602, 26.002) (-27.46, 25.8259) (-27.3033, 25.7017) (-27.1407, 25.5847) (-27.0236, 25.521) (-26.965, 25.4891) knots 0 0 0 0 0.125009 0.250019 0.375028 0.500033 0.625034 0.750027 0.812532 0.875036 0.937535 1 1 1 1 construction
  spline S26 degree 3 poles (-26.965, 25.4891) (-26.8774, 25.4542) (-26.746, 25.4019) (-26.5774, 25.3172) (-26.4558, 25.2449) (-26.3379, 25.1667) (-26.2277, 25.0778) (-26.1234, 24.9821) (-26.0302, 24.8754) (-25.9487, 24.7595) (-25.882, 24.6344) (-25.8324, 24.5016) (-25.8019, 24.363) (-25.7929, 24.2214) (-25.8055, 24.08) (-25.8426, 23.9432) (-25.8892, 23.8097) (-25.93, 23.6744) (-25.9803, 23.5419) (-26.0533, 23.42) (-26.1438, 23.3108) (-26.2499, 23.2166) (-26.3681, 23.1382) (-26.4956, 23.0763) (-26.6297, 23.0305) (-26.7678, 22.9989) (-26.9084, 22.9828) (-27.0498, 22.9756) (-27.1912, 22.9816) (-27.332, 22.9946) (-27.5182, 23.0252) (-27.6553, 23.0601) (-27.7467, 23.0834) knots 0 0 0 0 0.062498 0.093754 0.125008 0.156267 0.187517 0.21877 0.250029 0.281282 0.312529 0.343776 0.37503 0.406277 0.437515 0.468744 0.5 0.531256 0.562485 0.593723 0.62497 0.656224 0.687471 0.718718 0.749971 0.78123 0.812483 0.843733 0.874992 0.906246 0.937502 1 1 1 1 construction
  spline S27 degree 3 poles (-27.7467, 23.0834) (-27.8128, 23.092) (-27.945, 23.1093) (-28.1453, 23.1102) (-28.3451, 23.1019) (-28.6106, 23.0771) (-28.9402, 23.0257) (-29.3304, 22.9372) (-29.7146, 22.8258) (-30.0923, 22.6939) (-30.4637, 22.545) (-30.705, 22.4317) (-30.8257, 22.375) knots 0 0 0 0 0.062465 0.124964 0.187468 0.249973 0.374966 0.499967 0.624972 0.749981 0.874991 1 1 1 1 construction
  arc A6 (-30.8257, 22.375) -> (-30.9629, 21.0697) centre (-14, 19.9467) ccw construction
  spline S28 degree 3 poles (-30.9629, 21.0697) (-30.8566, 20.9892) (-30.6441, 20.8281) (-30.3118, 20.6053) (-29.9698, 20.3977) (-29.6171, 20.2089) (-29.2539, 20.0412) (-28.9422, 19.9224) (-28.6876, 19.8429) (-28.4939, 19.7932) (-28.2979, 19.7525) (-28.1649, 19.7419) (-28.0984, 19.7366) knots 0 0 0 0 0.125009 0.250019 0.375028 0.500033 0.625034 0.750027 0.812532 0.875036 0.937535 1 1 1 1 construction
  spline S29 degree 3 poles (-28.0984, 19.7366) (-28.0042, 19.7404) (-27.8629, 19.746) (-27.6744, 19.7372) (-27.5339, 19.7206) (-27.3944, 19.6971) (-27.2576, 19.6607) (-27.1234, 19.6157) (-26.9948, 19.5561) (-26.8733, 19.4834) (-26.7614, 19.3963) (-26.6621, 19.2951) (-26.5779, 19.1809) (-26.5121, 19.0552) (-26.466, 18.9209) (-26.4443, 18.7808) (-26.4325, 18.64) (-26.4147, 18.4998) (-26.4069, 18.3582) (-26.424, 18.2172) (-26.4622, 18.0806) (-26.5208, 17.9514) (-26.597, 17.8318) (-26.6883, 17.7233) (-26.7921, 17.6269) (-26.9054, 17.5419) (-27.0273, 17.47) (-27.1536, 17.4059) (-27.2852, 17.3539) (-27.4191, 17.3085) (-27.6017, 17.2607) (-27.7411, 17.2368) (-27.834, 17.2209) knots 0 0 0 0 0.062498 0.093754 0.125008 0.156267 0.187517 0.21877 0.250029 0.281282 0.312529 0.343776 0.37503 0.406277 0.437515 0.468744 0.5 0.531256 0.562485 0.593723 0.62497 0.656224 0.687471 0.718718 0.749971 0.78123 0.812483 0.843733 0.874992 0.906246 0.937502 1 1 1 1 construction
  spline S30 degree 3 poles (-27.834, 17.2209) (-27.8979, 17.2019) (-28.0258, 17.1639) (-28.2091, 17.0833) (-28.3882, 16.9944) (-28.6207, 16.8638) (-28.9009, 16.6828) (-29.2213, 16.4432) (-29.5271, 16.1852) (-29.8184, 15.9111) (-30.0972, 15.624) (-30.2715, 15.4223) (-30.3587, 15.3214) knots 0 0 0 0 0.062465 0.124964 0.187468 0.249973 0.374966 0.499967 0.624972 0.749981 0.874991 1 1 1 1 construction
  arc A7 (-30.3587, 15.3214) -> (-29.9531, 14.0732) centre (-14, 19.9467) ccw construction
  spline S31 degree 3 poles (-29.9531, 14.0732) (-29.8233, 14.0428) (-29.5637, 13.9821) (-29.1694, 13.9137) (-28.7726, 13.8632) (-28.3736, 13.8342) (-27.9735, 13.8287) (-27.6405, 13.8469) (-27.3756, 13.8779) (-27.1785, 13.9113) (-26.9827, 13.9538) (-26.857, 13.9982) (-26.7941, 14.0204) knots 0 0 0 0 0.125009 0.250019 0.375028 0.500033 0.625034 0.750027 0.812532 0.875036 0.937535 1 1 1 1 construction
  spline S32 degree 3 poles (-26.7941, 14.0204) (-26.7096, 14.0622) (-26.5827, 14.1248) (-26.407, 14.1935) (-26.2719, 14.2354) (-26.1349, 14.2707) (-25.9951, 14.2931) (-25.8542, 14.3066) (-25.7125, 14.3044) (-25.5719, 14.2874) (-25.4343, 14.2534) (-25.3024, 14.2013) (-25.179, 14.1312) (-25.0678, 14.0432) (-24.9711, 13.9392) (-24.8942, 13.8201) (-24.8262, 13.6962) (-24.7529, 13.5753) (-24.6882, 13.4492) (-24.6465, 13.3134) (-24.6258, 13.1731) (-24.6268, 13.0312) (-24.6477, 12.8909) (-24.687, 12.7547) (-24.7426, 12.6245) (-24.8116, 12.5007) (-24.8937, 12.3854) (-24.983, 12.2756) (-25.082, 12.1745) (-25.1859, 12.0785) (-25.3333, 11.9606) (-25.4509, 11.8821) (-25.5294, 11.8298) knots 0 0 0 0 0.062498 0.093754 0.125008 0.156267 0.187517 0.21877 0.250029 0.281282 0.312529 0.343776 0.37503 0.406277 0.437515 0.468744 0.5 0.531256 0.562485 0.593723 0.62497 0.656224 0.687471 0.718718 0.749971 0.78123 0.812483 0.843733 0.874992 0.906246 0.937502 1 1 1 1 construction
  spline S33 degree 3 poles (-25.5294, 11.8298) (-25.58, 11.7864) (-25.6814, 11.6997) (-25.816, 11.5515) (-25.9435, 11.3975) (-26.1028, 11.1835) (-26.2851, 10.9042) (-26.4804, 10.555) (-26.6548, 10.1949) (-26.8094, 9.826) (-26.9473, 9.4504) (-27.0245, 9.1952) (-27.0632, 9.0676) knots 0 0 0 0 0.062465 0.124964 0.187468 0.249973 0.374966 0.499967 0.624972 0.749981 0.874991 1 1 1 1 construction
  arc A8 (-27.0632, 9.0676) -> (-26.1849, 8.0922) centre (-14, 19.9467) ccw construction
  spline S34 degree 3 poles (-26.1849, 8.0922) (-26.054, 8.1173) (-25.7921, 8.1675) (-25.4042, 8.2653) (-25.0211, 8.3806) (-24.6447, 8.5164) (-24.277, 8.6741) (-23.9802, 8.8262) (-23.7508, 8.9622) (-23.5843, 9.0729) (-23.4228, 9.1914) (-23.326, 9.2831) (-23.2776, 9.3289) knots 0 0 0 0 0.125009 0.250019 0.375028 0.500033 0.625034 0.750027 0.812532 0.875036 0.937535 1 1 1 1 construction
  spline S35 degree 3 poles (-23.2776, 9.3289) (-23.2173, 9.4015) (-23.1269, 9.5103) (-22.9943, 9.6445) (-22.888, 9.7378) (-22.7771, 9.8257) (-22.6586, 9.903) (-22.5353, 9.9727) (-22.405, 10.0283) (-22.2696, 10.07) (-22.1301, 10.0948) (-21.9884, 10.101) (-21.8472, 10.0871) (-21.7098, 10.0519) (-21.5791, 9.9962) (-21.4604, 9.9187) (-21.3479, 9.8331) (-21.2318, 9.7525) (-21.1214, 9.6637) (-21.028, 9.5566) (-20.9521, 9.4368) (-20.8953, 9.3068) (-20.8573, 9.1701) (-20.8378, 9.0297) (-20.8357, 8.8881) (-20.8483, 8.747) (-20.8764, 8.6082) (-20.9133, 8.4716) (-20.9627, 8.339) (-21.0186, 8.209) (-21.1052, 8.0414) (-21.1808, 7.9218) (-21.2311, 7.8421) knots 0 0 0 0 0.062498 0.093754 0.125008 0.156267 0.187517 0.21877 0.250029 0.281282 0.312529 0.343776 0.37503 0.406277 0.437515 0.468744 0.5 0.531256 0.562485 0.593723 0.62497 0.656224 0.687471 0.718718 0.749971 0.78123 0.812483 0.843733 0.874992 0.906246 0.937502 1 1 1 1 construction
  spline S36 degree 3 poles (-21.2311, 7.8421) (-21.2598, 7.7819) (-21.3171, 7.6615) (-21.3799, 7.4713) (-21.4337, 7.2787) (-21.4921, 7.0185) (-21.5451, 6.6892) (-21.5815, 6.2908) (-21.5943, 5.8909) (-21.5855, 5.4909) (-21.5587, 5.0917) (-21.5255, 4.8272) (-21.5089, 4.6949) knots 0 0 0 0 0.062465 0.124964 0.187468 0.249973 0.374966 0.499967 0.624972 0.749981 0.874991 1 1 1 1 construction
  arc A9 (-21.5089, 4.6949) -> (-20.3099, 4.1611) centre (-14, 19.9467) ccw construction
  spline S37 degree 3 poles (-20.3099, 4.1611) (-20.2004, 4.2372) (-19.9816, 4.3895) (-19.667, 4.6367) (-19.3639, 4.8978) (-19.0753, 5.1749) (-18.8036, 5.4686) (-18.5943, 5.7283) (-18.44, 5.9459) (-18.3329, 6.1147) (-18.2336, 6.2886) (-18.1824, 6.4118) (-18.1569, 6.4733) knots 0 0 0 0 0.125009 0.250019 0.375028 0.500033 0.625034 0.750027 0.812532 0.875036 0.937535 1 1 1 1 construction
  spline S38 degree 3 poles (-18.1569, 6.4733) (-18.1313, 6.5641) (-18.093, 6.7003) (-18.0264, 6.8768) (-17.9672, 7.0053) (-17.9017, 7.1308) (-17.8249, 7.2496) (-17.7406, 7.3633) (-17.6442, 7.4672) (-17.5375, 7.5603) (-17.4201, 7.6398) (-17.2931, 7.703) (-17.1585, 7.7478) (-17.0186, 7.7715) (-16.8766, 7.7738) (-16.7367, 7.7512) (-16.5991, 7.7188) (-16.4603, 7.6924) (-16.3232, 7.6562) (-16.1944, 7.5963) (-16.0763, 7.5177) (-15.9715, 7.4221) (-15.8813, 7.3127) (-15.8063, 7.1924) (-15.7467, 7.0638) (-15.7009, 6.9298) (-15.6702, 6.7916) (-15.6483, 6.6518) (-15.6395, 6.5105) (-15.6377, 6.3691) (-15.6487, 6.1807) (-15.669, 6.0407) (-15.6826, 5.9474) knots 0 0 0 0 0.062498 0.093754 0.125008 0.156267 0.187517 0.21877 0.250029 0.281282 0.312529 0.343776 0.37503 0.406277 0.437515 0.468744 0.5 0.531256 0.562485 0.593723 0.62497 0.656224 0.687471 0.718718 0.749971 0.78123 0.812483 0.843733 0.874992 0.906246 0.937502 1 1 1 1 construction
  spline S39 degree 3 poles (-15.6826, 5.9474) (-15.6843, 5.8808) (-15.6877, 5.7474) (-15.6676, 5.5482) (-15.6385, 5.3504) (-15.586, 5.0889) (-15.5005, 4.7665) (-15.3717, 4.3877) (-15.2207, 4.0172) (-15.0501, 3.6554) (-14.8632, 3.3016) (-14.7252, 3.0734) (-14.6562, 2.9593) knots 0 0 0 0 0.062465 0.124964 0.187468 0.249973 0.374966 0.499967 0.624972 0.749981 0.874991 1 1 1 1 construction
  arc A10 (-14.6562, 2.9593) -> (-13.3438, 2.9593) centre (-14, 19.9467) ccw construction
  spline S40 degree 3 poles (-13.3438, 2.9593) (-13.2748, 3.0734) (-13.1368, 3.3016) (-12.9499, 3.6554) (-12.7793, 4.0172) (-12.6283, 4.3877) (-12.4995, 4.7665) (-12.414, 5.0889) (-12.3615, 5.3504) (-12.3324, 5.5482) (-12.3123, 5.7474) (-12.3157, 5.8808) (-12.3174, 5.9474) knots 0 0 0 0 0.125009 0.250019 0.375028 0.500033 0.625034 0.750027 0.812532 0.875036 0.937535 1 1 1 1 construction
  spline S41 degree 3 poles (-12.3174, 5.9474) (-12.331, 6.0407) (-12.3513, 6.1807) (-12.3623, 6.3691) (-12.3605, 6.5105) (-12.3517, 6.6518) (-12.3298, 6.7916) (-12.2991, 6.9298) (-12.2533, 7.0638) (-12.1937, 7.1924) (-12.1187, 7.3127) (-12.0285, 7.4221) (-11.9237, 7.5177) (-11.8056, 7.5963) (-11.6768, 7.6562) (-11.5397, 7.6924) (-11.4009, 7.7188) (-11.2633, 7.7512) (-11.1234, 7.7738) (-10.9814, 7.7715) (-10.8415, 7.7478) (-10.7069, 7.703) (-10.5799, 7.6398) (-10.4625, 7.5603) (-10.3558, 7.4672) (-10.2594, 7.3633) (-10.1751, 7.2496) (-10.0983, 7.1308) (-10.0328, 7.0053) (-9.9736, 6.8768) (-9.907, 6.7003) (-9.8687, 6.5641) (-9.8431, 6.4733) knots 0 0 0 0 0.062498 0.093754 0.125008 0.156267 0.187517 0.21877 0.250029 0.281282 0.312529 0.343776 0.37503 0.406277 0.437515 0.468744 0.5 0.531256 0.562485 0.593723 0.62497 0.656224 0.687471 0.718718 0.749971 0.78123 0.812483 0.843733 0.874992 0.906246 0.937502 1 1 1 1 construction
  spline S42 degree 3 poles (-9.8431, 6.4733) (-9.8176, 6.4118) (-9.7664, 6.2886) (-9.6671, 6.1147) (-9.56, 5.9459) (-9.4057, 5.7283) (-9.1964, 5.4686) (-8.9247, 5.1749) (-8.6361, 4.8978) (-8.333, 4.6367) (-8.0184, 4.3895) (-7.7996, 4.2372) (-7.6901, 4.1611) knots 0 0 0 0 0.062465 0.124964 0.187468 0.249973 0.374966 0.499967 0.624972 0.749981 0.874991 1 1 1 1 construction
  arc A11 (-7.6901, 4.1611) -> (-6.4911, 4.6949) centre (-14, 19.9467) ccw construction
  spline S43 degree 3 poles (-6.4911, 4.6949) (-6.4745, 4.8272) (-6.4413, 5.0917) (-6.4145, 5.4909) (-6.4057, 5.8909) (-6.4185, 6.2908) (-6.4549, 6.6892) (-6.5079, 7.0185) (-6.5663, 7.2787) (-6.6201, 7.4713) (-6.6829, 7.6615) (-6.7402, 7.7819) (-6.7689, 7.8421) knots 0 0 0 0 0.125009 0.250019 0.375028 0.500033 0.625034 0.750027 0.812532 0.875036 0.937535 1 1 1 1 construction
  spline S44 degree 3 poles (-6.7689, 7.8421) (-6.8192, 7.9218) (-6.8948, 8.0414) (-6.9814, 8.209) (-7.0373, 8.339) (-7.0867, 8.4716) (-7.1236, 8.6082) (-7.1517, 8.747) (-7.1643, 8.8881) (-7.1622, 9.0297) (-7.1427, 9.1701) (-7.1047, 9.3068) (-7.0479, 9.4368) (-6.972, 9.5566) (-6.8786, 9.6637) (-6.7682, 9.7525) (-6.6521, 9.8331) (-6.5396, 9.9187) (-6.4209, 9.9962) (-6.2902, 10.0519) (-6.1528, 10.0871) (-6.0116, 10.101) (-5.8699, 10.0948) (-5.7304, 10.07) (-5.595, 10.0283) (-5.4647, 9.9727) (-5.3414, 9.903) (-5.2229, 9.8257) (-5.112, 9.7378) (-5.0057, 9.6445) (-4.8731, 9.5103) (-4.7827, 9.4015) (-4.7224, 9.3289) knots 0 0 0 0 0.062498 0.093754 0.125008 0.156267 0.187517 0.21877 0.250029 0.281282 0.312529 0.343776 0.37503 0.406277 0.437515 0.468744 0.5 0.531256 0.562485 0.593723 0.62497 0.656224 0.687471 0.718718 0.749971 0.78123 0.812483 0.843733 0.874992 0.906246 0.937502 1 1 1 1 construction
  spline S45 degree 3 poles (-4.7224, 9.3289) (-4.674, 9.2831) (-4.5772, 9.1914) (-4.4157, 9.0729) (-4.2492, 8.9622) (-4.0198, 8.8262) (-3.723, 8.6741) (-3.3553, 8.5164) (-2.9789, 8.3806) (-2.5958, 8.2653) (-2.2079, 8.1675) (-1.946, 8.1173) (-1.8151, 8.0922) knots 0 0 0 0 0.062465 0.124964 0.187468 0.249973 0.374966 0.499967 0.624972 0.749981 0.874991 1 1 1 1 construction
  arc A12 (-1.8151, 8.0922) -> (-0.9368, 9.0676) centre (-14, 19.9467) ccw construction
  spline S46 degree 3 poles (-0.9368, 9.0676) (-0.9755, 9.1952) (-1.0527, 9.4504) (-1.1906, 9.826) (-1.3452, 10.1949) (-1.5196, 10.555) (-1.7149, 10.9042) (-1.8972, 11.1835) (-2.0565, 11.3975) (-2.184, 11.5515) (-2.3186, 11.6997) (-2.42, 11.7864) (-2.4706, 11.8298) knots 0 0 0 0 0.125009 0.250019 0.375028 0.500033 0.625034 0.750027 0.812532 0.875036 0.937535 1 1 1 1 construction
  spline S47 degree 3 poles (-2.4706, 11.8298) (-2.5491, 11.8821) (-2.6667, 11.9606) (-2.8141, 12.0785) (-2.918, 12.1745) (-3.017, 12.2756) (-3.1063, 12.3854) (-3.1884, 12.5007) (-3.2574, 12.6245) (-3.313, 12.7547) (-3.3523, 12.8909) (-3.3732, 13.0312) (-3.3742, 13.1731) (-3.3535, 13.3134) (-3.3118, 13.4492) (-3.2471, 13.5753) (-3.1738, 13.6962) (-3.1058, 13.8201) (-3.0289, 13.9392) (-2.9322, 14.0432) (-2.821, 14.1312) (-2.6976, 14.2013) (-2.5657, 14.2534) (-2.4281, 14.2874) (-2.2875, 14.3044) (-2.1458, 14.3066) (-2.0049, 14.2931) (-1.8651, 14.2707) (-1.7281, 14.2354) (-1.593, 14.1935) (-1.4173, 14.1248) (-1.2904, 14.0622) (-1.2059, 14.0204) knots 0 0 0 0 0.062498 0.093754 0.125008 0.156267 0.187517 0.21877 0.250029 0.281282 0.312529 0.343776 0.37503 0.406277 0.437515 0.468744 0.5 0.531256 0.562485 0.593723 0.62497 0.656224 0.687471 0.718718 0.749971 0.78123 0.812483 0.843733 0.874992 0.906246 0.937502 1 1 1 1 construction
  spline S48 degree 3 poles (-1.2059, 14.0204) (-1.143, 13.9982) (-1.0173, 13.9538) (-0.8215, 13.9113) (-0.6244, 13.8779) (-0.3595, 13.8469) (-0.0265, 13.8287) (0.3736, 13.8342) (0.7726, 13.8632) (1.1694, 13.9137) (1.5637, 13.9821) (1.8233, 14.0428) (1.9531, 14.0732) knots 0 0 0 0 0.062465 0.124964 0.187468 0.249973 0.374966 0.499967 0.624972 0.749981 0.874991 1 1 1 1 construction
  arc A13 (1.9531, 14.0732) -> (2.3587, 15.3214) centre (-14, 19.9467) ccw construction
  spline S49 degree 3 poles (2.3587, 15.3214) (2.2715, 15.4223) (2.0972, 15.624) (1.8184, 15.9111) (1.5271, 16.1852) (1.2213, 16.4432) (0.9009, 16.6828) (0.6207, 16.8638) (0.3882, 16.9944) (0.2091, 17.0833) (0.0258, 17.1639) (-0.1021, 17.2019) (-0.166, 17.2209) knots 0 0 0 0 0.125009 0.250019 0.375028 0.500033 0.625034 0.750027 0.812532 0.875036 0.937535 1 1 1 1 construction
  spline S50 degree 3 poles (-0.166, 17.2209) (-0.2589, 17.2368) (-0.3983, 17.2607) (-0.5809, 17.3085) (-0.7148, 17.3539) (-0.8464, 17.4059) (-0.9727, 17.47) (-1.0946, 17.5419) (-1.2079, 17.6269) (-1.3117, 17.7233) (-1.403, 17.8318) (-1.4792, 17.9514) (-1.5378, 18.0806) (-1.576, 18.2172) (-1.5931, 18.3582) (-1.5853, 18.4998) (-1.5675, 18.64) (-1.5557, 18.7808) (-1.534, 18.9209) (-1.4879, 19.0552) (-1.4221, 19.1809) (-1.3379, 19.2951) (-1.2386, 19.3963) (-1.1267, 19.4834) (-1.0052, 19.5561) (-0.8766, 19.6157) (-0.7424, 19.6607) (-0.6056, 19.6971) (-0.4661, 19.7206) (-0.3256, 19.7372) (-0.1371, 19.746) (0.0042, 19.7404) (0.0984, 19.7366) knots 0 0 0 0 0.062498 0.093754 0.125008 0.156267 0.187517 0.21877 0.250029 0.281282 0.312529 0.343776 0.37503 0.406277 0.437515 0.468744 0.5 0.531256 0.562485 0.593723 0.62497 0.656224 0.687471 0.718718 0.749971 0.78123 0.812483 0.843733 0.874992 0.906246 0.937502 1 1 1 1 construction